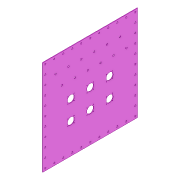
# Autodesk Inventor part: RD-A001-P001-REV0-noCutouts
Saved by Autodesk Inventor 2017 (Build 210142000, 142)
## iProperties
Created: 2017-05-03
Part Number: RD-A001-P001-REV0-noCutouts
Material: Generic
Document SubType Name: Modeling
Designer: Kathryn Rosie
Density: 1 g/cm^3
Appearance: Default(2)
Author: Kathryn Rosie
Autodesk Inventor part; units mm, degrees
ref_plane "YZ Plane" through (0, 0, 0) normal (1, 0, 0) x (0, 1, 0)
ref_plane "XZ Plane" through (0, 0, 0) normal (0, 1, 0) x (-1, 0, 0)
ref_plane "XY Plane" through (0, 0, 0) normal (0, 0, 1) x (1, 0, 0)
sketch "Sketch4" plane through (0, 0, 0) normal (1, 0, 0) x (0, 1, 0)
  line L0 (-187, 187) -> (187, 187)
  line L1 (187, 187) -> (187, -187)
  line L2 (187, -187) -> (-187, -187)
  line L3 (-187, -187) -> (-187, 187)
  line L4 (-187, 187) -> (187, -187) construction
  line L5 (187, 187) -> (-187, -187) construction
  arc A0 (121.76, 139.7462) -> (125.24, 139.7462) centre (123.5, 137) ccw
  line L6 (125.24, 139.7462) -> (121.76, 139.7462)
  line L7 (125.24, 88.9462) -> (121.76, 88.9462)
  arc A1 (121.76, 88.9462) -> (125.24, 88.9462) centre (123.5, 86.2) ccw
  line L8 (125.24, 38.1462) -> (121.76, 38.1462)
  arc A2 (121.76, 38.1462) -> (125.24, 38.1462) centre (123.5, 35.4) ccw
  line L9 (125.24, -12.6538) -> (121.76, -12.6538)
  arc A3 (121.76, -12.6538) -> (125.24, -12.6538) centre (123.5, -15.4) ccw
  line L10 (125.24, -63.4538) -> (121.76, -63.4538)
  arc A4 (121.76, -63.4538) -> (125.24, -63.4538) centre (123.5, -66.2) ccw
  line L11 (125.24, -114.2538) -> (121.76, -114.2538)
  arc A5 (121.76, -114.2538) -> (125.24, -114.2538) centre (123.5, -117) ccw
  arc A6 (70.96, 114.3462) -> (74.44, 114.3462) centre (72.7, 111.6) ccw
  line L12 (74.44, 114.3462) -> (70.96, 114.3462)
  line L13 (74.44, 63.5462) -> (70.96, 63.5462)
  arc A7 (70.96, 63.5462) -> (74.44, 63.5462) centre (72.7, 60.8) ccw
  line L14 (74.44, 12.7462) -> (70.96, 12.7462)
  arc A8 (70.96, 12.7462) -> (74.44, 12.7462) centre (72.7, 10) ccw
  line L15 (74.44, -38.0538) -> (70.96, -38.0538)
  arc A9 (70.96, -38.0538) -> (74.44, -38.0538) centre (72.7, -40.8) ccw
  line L16 (74.44, -88.8538) -> (70.96, -88.8538)
  arc A10 (70.96, -88.8538) -> (74.44, -88.8538) centre (72.7, -91.6) ccw
  line L17 (74.44, -139.6538) -> (70.96, -139.6538)
  arc A11 (70.96, -139.6538) -> (74.44, -139.6538) centre (72.7, -142.4) ccw
  circle A12 centre (9.2, 76.205) radius 14
  circle A13 centre (9.2, 0.005) radius 14
  circle A14 centre (9.2, -76.195) radius 14
  circle A15 centre (-67, 0.005) radius 14
  circle A16 centre (-67, -76.195) radius 14
  circle A17 centre (-67, 76.205) radius 14
  point P0 (0, 0)
  point P1 (177.5, 177.5)
  point P2 (177.5, 142)
  point P3 (177.5, 106.5)
  point P4 (177.5, 71)
  point P5 (177.5, 35.5)
  point P6 (177.5, 0)
  point P7 (177.5, -35.5)
  point P8 (177.5, -71)
  point P9 (177.5, -106.5)
  point P10 (177.5, -142)
  point P11 (177.5, -177.5)
  point P12 (142, 177.5)
  point P13 (106.5, 177.5)
  point P14 (71, 177.5)
  point P15 (35.5, 177.5)
  point P16 (0, 177.5)
  point P17 (-35.5, 177.5)
  point P18 (-71, 177.5)
  point P19 (-106.5, 177.5)
  point P20 (-142, 177.5)
  point P21 (-177.5, 177.5)
  point P22 (142, -177.5)
  point P23 (106.5, -177.5)
  point P24 (71, -177.5)
  point P25 (35.5, -177.5)
  point P26 (0, -177.5)
  point P27 (-35.5, -177.5)
  point P28 (-71, -177.5)
  point P29 (-106.5, -177.5)
  point P30 (-142, -177.5)
  point P31 (-177.5, -177.5)
  point P32 (-177.5, 142)
  point P33 (-177.5, 106.5)
  point P34 (-177.5, 71)
  point P35 (-177.5, 35.5)
  point P36 (-177.5, 0)
  point P37 (-177.5, -35.5)
  point P38 (-177.5, -71)
  point P39 (-177.5, -106.5)
  point P40 (-177.5, -142)
  dimension "d34" = 374
  dimension "d35" = 374
  dimension "d36" = 9.5
  dimension "d39" = 35.5
  dimension "d46" = 35.5
  dimension "d53" = 35.5
  dimension "d60" = 35.5
  dimension "d65" = 6.502
  dimension "d66" = 50
  dimension "d67" = 63.5
  dimension "d68" = 3.48
  dimension "d71" = 50.8
  dimension "d96" = 6.502
  dimension "d97" = 3.48
  dimension "d98" = 25.4
  dimension "d99" = 50.8
  dimension "d102" = 50.8
  dimension "d107" = 28
  dimension "d110" = 76.2
  dimension "d115" = 110.795
  dimension "d116" = 177.8
  dimension "d119" = 76.2
  constraints: 36 end point, 24 point on circle, 18 centre point, 6 horizontal, 5 vertical, 2 midpoint, 2 parallel, 1 perpendicular, 1 point on line, 99 other
  measures "d34" distance of L1.end L2.end
  measures "d35" distance of L0.end L1.end
  measures "d36" distance from line of L1 point (177.5, 177.5)
  measures "d39" distance of point (177.5, 177.5) point (177.5, 142)
  measures "d46" distance of point (177.5, 177.5) point (142, 177.5)
  measures "d53" distance of point (177.5, -177.5) point (142, -177.5)
  measures "d60" distance of point (-177.5, 177.5) point (-177.5, 142)
  measures "d65" diameter of A0
  measures "d66" distance from line of L0 A0.centre
  measures "d67" distance from line of L1 A0.centre
  measures "d68" distance of L6.start L6.end
  measures "d71" distance of L6.start L7.start
  measures "d96" diameter of A6
  measures "d97" distance of L12.start L12.end
  measures "d98" vertical distance of A6.centre A0.centre
  measures "d99" horizontal distance of A0.centre A6.centre
  measures "d102" distance of L12.start L13.start
  measures "d107" diameter of A12
  measures "d110" distance of A12.centre A13.centre
  measures "d115" distance from line of L0 A12.centre
  measures "d116" distance from line of L1 A12.centre
  measures "d119" distance of A13.centre A15.centre
extrude "Extrusion3" add sketch "Sketch4" along normal blind 2
hole "Hole1" at (0, 177.5, 177.5) at (0, 177.5, 142) at (0, 177.5, 106.5) at (0, 177.5, 71) at (0, 177.5, 35.5) at (0, 177.5, 0) at (0, 177.5, -35.5) at (0, 177.5, -71) at (0, 177.5, -106.5) at (0, 177.5, -142) at (0, 177.5, -177.5) at (0, 142, 177.5) at (0, 106.5, 177.5) at (0, 71, 177.5) at (0, 35.5, 177.5) at (0, 0, 177.5) at (0, -35.5, 177.5) at (0, -71, 177.5) at (0, -106.5, 177.5) at (0, -142, 177.5) at (0, -177.5, 177.5) at (0, 142, -177.5) at (0, 106.5, -177.5) at (0, 71, -177.5) at (0, 35.5, -177.5) at (0, 0, -177.5) at (0, -35.5, -177.5) at (0, -71, -177.5) at (0, -106.5, -177.5) at (0, -142, -177.5) at (0, -177.5, -177.5) at (0, -177.5, 142) at (0, -177.5, 106.5) at (0, -177.5, 71) at (0, -177.5, 35.5) at (0, -177.5, 0) at (0, -177.5, -35.5) at (0, -177.5, -71) at (0, -177.5, -106.5) at (0, -177.5, -142) direction (1, 0, 0) diameter 6.2 end through all
sketch "Sketch5" plane through (2, 0, 0) normal (1, 0, 0) x (0, 0, -1)
  circle A0 centre (-76.205, 9.2) radius 14 projected
  circle A1 centre (-0.005, 9.2) radius 14 projected
  circle A2 centre (76.195, 9.2) radius 14 projected
  circle A3 centre (76.195, -67) radius 14 projected
  circle A4 centre (-0.005, -67) radius 14 projected
  circle A5 centre (-76.205, -67) radius 14 projected
  circle A6 centre (-76.205, 9.2) radius 17.5 construction
  circle A7 centre (-0.005, 9.2) radius 17.5 construction
  circle A8 centre (76.195, 9.2) radius 17.5 construction
  circle A9 centre (76.195, -67) radius 17.5 construction
  circle A10 centre (-0.005, -67) radius 17.5 construction
  circle A11 centre (-76.205, -67) radius 17.5 construction
  line L0 (-76.205, 9.2) -> (-63.8306, 21.5744) construction
  line L1 (-76.205, 9.2) -> (-58.705, 9.2) construction
  line L2 (-0.005, 9.2) -> (12.3694, 21.5744) construction
  line L3 (-0.005, 9.2) -> (17.495, 9.2) construction
  line L4 (76.195, 9.2) -> (88.5694, 21.5744) construction
  line L5 (76.195, 9.2) -> (93.695, 9.2) construction
  line L6 (76.195, -67) -> (88.5694, -54.6256) construction
  line L7 (76.195, -67) -> (93.695, -67) construction
  line L8 (-0.005, -67) -> (12.3694, -54.6256) construction
  line L9 (-0.005, -67) -> (17.495, -67) construction
  line L10 (-76.205, -67) -> (-63.8306, -54.6256) construction
  line L11 (-76.205, -67) -> (-58.705, -67) construction
  circle A12 centre (-63.8306, 21.5744) radius 1.25
  circle A13 centre (12.3694, 21.5744) radius 1.25
  circle A14 centre (88.5694, 21.5744) radius 1.25
  circle A15 centre (88.5694, -54.6256) radius 1.25
  circle A16 centre (12.3694, -54.6256) radius 1.25
  circle A17 centre (-63.8306, -54.6256) radius 1.25
  circle A18 centre (-88.5794, 21.5744) radius 1.25
  circle A19 centre (-88.5794, -3.1744) radius 1.25
  circle A20 centre (-63.8306, -3.1744) radius 1.25
  circle A21 centre (-12.3794, 21.5744) radius 1.25
  circle A22 centre (-12.3794, -3.1744) radius 1.25
  circle A23 centre (12.3694, -3.1744) radius 1.25
  circle A24 centre (63.8206, 21.5744) radius 1.25
  circle A25 centre (63.8206, -3.1744) radius 1.25
  circle A26 centre (88.5694, -3.1744) radius 1.25
  circle A27 centre (63.8206, -54.6256) radius 1.25
  circle A28 centre (63.8206, -79.3744) radius 1.25
  circle A29 centre (88.5694, -79.3744) radius 1.25
  circle A30 centre (-12.3794, -54.6256) radius 1.25
  circle A31 centre (-12.3794, -79.3744) radius 1.25
  circle A32 centre (12.3694, -79.3744) radius 1.25
  circle A33 centre (-88.5794, -54.6256) radius 1.25
  circle A34 centre (-88.5794, -79.3744) radius 1.25
  circle A35 centre (-63.8306, -79.3744) radius 1.25
  point P0 (0, 0)
  dimension "d133" = 35
  dimension "d134" = 35
  dimension "d135" = 35
  dimension "d136" = 35
  dimension "d137" = 35
  dimension "d138" = 35
  dimension "d139" = 45
  dimension "d140" = 45
  dimension "d141" = 45
  dimension "d142" = 45
  dimension "d143" = 45
  dimension "d144" = 45
  dimension "d145" = 2.5
  dimension "d146" = 2.5
  dimension "d147" = 2.5
  dimension "d148" = 2.5
  dimension "d149" = 2.5
  dimension "d150" = 2.5
  dimension "d153" = 360
  dimension "d157" = 360
  dimension "d161" = 360
  dimension "d165" = 360
  dimension "d169" = 360
  dimension "d173" = 360
  constraints: 24 centre point, 24 end point, 12 coincident, 6 equal length, 6 horizontal, 72 other
  measures "d139" angle of L1 L0
  measures "d140" angle of L3 L2
  measures "d141" angle of L5 L4
  measures "d142" angle of L7 L6
  measures "d143" angle of L9 L8
  measures "d144" angle of L11 L10
  measures "d145" diameter of A12
  measures "d146" diameter of A13
  measures "d147" diameter of A14
  measures "d148" diameter of A15
  measures "d149" diameter of A16
  measures "d150" diameter of A17
extrude "Extrusion4" cut sketch "Sketch5" against normal up to surface (2 mm away) contours A12 | A13 | A14 | A15 | A16 | A17 | A18 | A19 | A20 | A21 | A22 | A23 | A24 | A25 | A26 | A27 | A28 | A29 | A30 | A31 | A32 | A33 | A34 | A35
body "Solid4"
